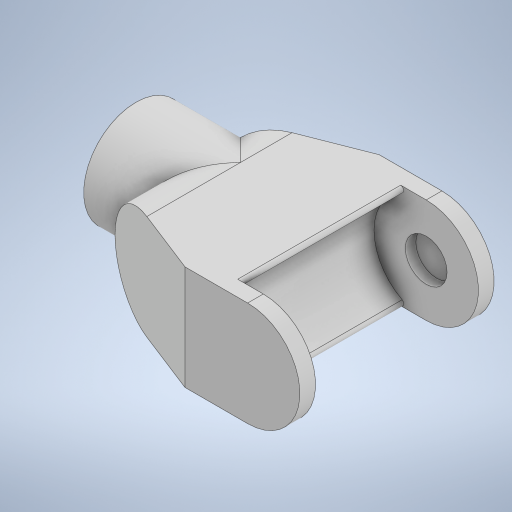
# Autodesk Inventor part: Arm 5 v0.1
Saved by Autodesk Inventor 2023 (Build 270158000, 158)
## iProperties
Created: 2024-06-24
Part Number: Arm 5 v0.1
Material: Generic
Document SubType Name: Modeling
Designer: Swoby
Density: 1 g/cm^3
Appearance: Default
Author: Swoby
Autodesk Inventor part; units mm, degrees
ref_plane "XZ Plane" through (0, 0, 0) normal (0, 1, 0) x (-1, 0, 0)
ref_plane "XY Plane" through (0, 0, 0) normal (0, 0, 1) x (1, 0, 0)
sketch "Sketch1" plane through (0, 0, 0) normal (0, 0, 1) x (1, 0, 0)
  circle A0 centre (0, 0) radius 25
  line L0 (0, 25) -> (-60, 25)
  line L1 (0, -25) -> (-60, -25)
  arc A1 (-60, 25) -> (-60, -25) centre (-60, 0) ccw
  dimension "d0" = 50
  dimension "d1" = 60
  dimension "d2" = 60
  dimension "d3" = 25
  constraints: 4 end point, 4 point on circle, 2 centre point, 2 horizontal, 2 tangent, 1 coincident
  measures "d0" diameter of A0
  measures "d1" distance of L0.start L0.end
  measures "d2" distance of L1.start L1.end
  measures "d3" radius of A1
extrude "Extrusion1" add sketch "Sketch1" along normal mid plane 93
sketch "Sketch2" plane through (0, 0, 0) normal (0, 0, 1) x (1, 0, 0)
  arc A0 (0, -25) -> (0, 25) centre (0, 0) ccw
  arc A1 (-12.2474, 25) -> (-11.5542, 22.1698) centre (-12.2474, 23.5) ccw construction
  arc A2 (-11.5542, -22.1698) -> (-12.2474, -25) centre (-12.2474, -23.5) ccw construction
  line L0 (0, -25) -> (-60, -25) projected
  line L1 (-60, 25) -> (0, 25) projected
  line L2 (-12.2474, 25) -> (0, 25)
  arc A3 (0, -25) -> (0, 25) centre (0, 0) ccw projected
  line L3 (-12.2474, -25) -> (0, -25)
  arc A4 (-11.5542, -22.1698) -> (0, -25) centre (0, 0) ccw construction
  arc A5 (-12.2474, -25) -> (-11.5542, -22.1698) centre (-12.2474, -23.5) ccw
  arc A6 (-11.5542, 22.1698) -> (-12.2474, 25) centre (-12.2474, 23.5) ccw
  arc A7 (-11.5542, 22.1698) -> (-11.5542, -22.1698) centre (0, 0) ccw
  arc A8 (0, 25) -> (-11.5542, 22.1698) centre (0, 0) ccw construction
  dimension "d7" = 3
  dimension "d8" = 3
  constraints: 16 point on circle, 8 centre point, 5 end point, 5 tangent, 2 point on line, 1 coincident
  measures "d7" diameter of A1
  measures "d8" diameter of A2
extrude "Extrusion2" cut sketch "Sketch2" along normal mid plane 78
sketch "Sketch3" plane through (0, 0, 0) normal (0, 0, 1) x (1, 0, 0)
  circle A0 centre (0, 0) radius 10
  dimension "d11" = 20
  constraints: 1 centre point, 1 coincident
  measures "d11" diameter of A0
extrude "Extrusion3" cut sketch "Sketch3" along normal mid plane 88
sketch "Sketch4" plane through (-60, 25, -46.5) normal (0, 1, 0) x (1, 0, 0)
  line L0 (35, -7.5) -> (35, -85.5) projected
  line L1 (0, -93) -> (60, -93) projected
  line L2 (30, -93) -> (30, 0)
  line L3 (60, 0) -> (0, 0) projected
  line L4 (30, -93) -> (-25, -71.5)
  line L5 (-25, 0) -> (-25, -93) projected
  line L6 (-25, -71.5) -> (-25, -93)
  line L7 (30, -93) -> (-25, -93)
  line L8 (30, 0) -> (-25, -21.5)
  line L9 (-25, 0) -> (30, 0)
  line L10 (-25, -21.5) -> (-25, 0)
  point P0 (60, -46.5)
  dimension "d14" = 5
  dimension "d15" = 50
  dimension "d16" = 21.5
  constraints: 14 end point, 2 collinear, 2 midpoint, 2 point on line, 2 vertical, 1 perpendicular
  measures "d14" distance between parallel lines of L0 L2
  measures "d15" distance of L8.end L4.end
  measures "d16" distance of L5.end L4.end
extrude "Extrusion4" cut sketch "Sketch4" against normal through all contours L7 L5 L4 L1 | L8 L5 L9 L3
ref_plane "Work Plane1" through (-60, 0, 0) normal (1, 0, 0) x (0, 1, 0)
sketch "Sketch5" plane through (-60, 0, 0) normal (1, 0, 0) x (0, 1, 0)
  circle A0 centre (0, -10) radius 25
  line L0 (-25, -46.5) -> (25, -46.5) projected
  line L1 (0, -46.5) -> (0, -10)
  dimension "d20" = 50
  dimension "d23" = 36.5
  constraints: 2 end point, 1 centre point, 1 coincident, 1 midpoint, 1 vertical
  measures "d20" diameter of A0
  measures "d23" distance from line of L0 point (0, -10)
extrude "Extrusion5" add sketch "Sketch5" against normal blind 50
body "Solid1"
